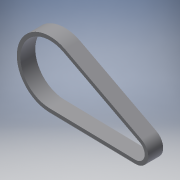
# Autodesk Inventor part: Short First Stage Belt
Saved by Autodesk Inventor 2019.4 (Build 234330000, 330)
## iProperties
Created: 2020-01-22
Part Number: Short First Stage Belt
Material: Rubber
Document SubType Name: Modeling
Designer: Mark
Mass: 15.9119 g
Surface Area: 117.866 cm^2
Volume: 17.1096 cm^3
Density: 0.93 g/cm^3
Appearance: Rubber - Black
Author: Mark
Autodesk Inventor part; units mm, degrees
ref_plane "YZ Plane" through (0, 0, 0) normal (1, 0, 0) x (0, 1, 0)
ref_plane "XZ Plane" through (0, 0, 0) normal (0, 1, 0) x (-1, 0, 0)
ref_plane "XY Plane" through (0, 0, 0) normal (0, 0, 1) x (1, 0, 0)
sketch "Sketch1" plane through (0, 0, 0) normal (0, 0, 1) x (1, 0, 0)
  arc A0 (-0.2263, -11.4028) -> (5.2912, 10.1033) centre (0, 0) ccw
  arc A1 (-71.5378, 50.3394) -> (-86.9366, -9.6815) centre (-86.3049, 22.1422) ccw
  line L0 (0, 0) -> (-86.3049, 22.1422)
  line L1 (-86.9366, -9.6815) -> (-0.2263, -11.4028)
  line L2 (-71.5378, 50.3394) -> (5.2912, 10.1033)
  arc A2 (-0.2561, -12.9025) -> (5.9871, 11.4321) centre (0, 0) ccw
  line L3 (-0.2561, -12.9025) -> (-86.9664, -11.1812)
  arc A3 (-70.8418, 51.6682) -> (-86.9664, -11.1812) centre (-86.3049, 22.1422) ccw
  line L4 (-70.8418, 51.6682) -> (5.9871, 11.4321)
  line L5 (-0.1847, -9.3032) -> (-86.8949, -7.5819)
  arc A4 (-72.512, 48.4791) -> (-86.8949, -7.5819) centre (-86.3049, 22.1422) ccw
  line L6 (-72.512, 48.4791) -> (4.3169, 8.243)
  arc A5 (-0.1847, -9.3032) -> (4.3169, 8.243) centre (0, 0) ccw
  dimension "d0" = 22.81
  dimension "d1" = 63.66
  dimension "d2" = 89.1
  dimension "d3" = 1.5
  dimension "d4" = 2.1
  constraints: 14 end point, 12 point on circle, 6 centre point, 4 tangent, 2 coincident, 6 other
  measures "d0" diameter of A0
  measures "d1" diameter of A1
  measures "d2" distance of L0.start L0.end
  measures "d3" distance between parallel lines of L2 L4
  measures "d4" distance between parallel lines of L1 L5
extrude "Extrusion1" add sketch "Sketch1" along normal blind 15 contours L1 A1 L2 A0 | L3 A3 L4 A2
body "Solid1"
